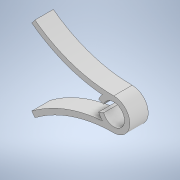
# Autodesk Inventor part: 8mmClamp
Saved by Autodesk Inventor 2020.2 (Build 242310000, 310)
## iProperties
Created: 2020-08-26
Part Number: 8mmClamp
Material: Generic
Document SubType Name: Modeling
Designer: elmar
Density: 1 g/cm^3
Appearance: Default
Author: elmar
Autodesk Inventor part; units mm, degrees
ref_plane "YZ Plane" through (0, 0, 0) normal (1, 0, 0) x (0, 1, 0)
ref_plane "XZ Plane" through (0, 0, 0) normal (0, 1, 0) x (-1, 0, 0)
ref_plane "XY Plane" through (0, 0, 0) normal (0, 0, 1) x (1, 0, 0)
sketch "Sketch1" plane through (0, 0, 0) normal (0, 0, 1) x (1, 0, 0)
  circle A0 centre (0, 0) radius 4.1
  circle A1 centre (0, 0) radius 6.1
  arc A2 (-30, 16.1) -> (0, 6.1) centre (0, 56.1) ccw
  line L0 (0, -78.54) -> (0, 78.54) projected
  arc A3 (-31.2, 14.5) -> (0, 4.1) centre (0, 56.1) ccw
  line L1 (-30, 16.1) -> (-31.2, 14.5)
  line L2 (-39.6726, 0) -> (13.7288, 0) projected
  arc A4 (0, -6.1) -> (-30, -16.1) centre (0, -56.1) ccw
  arc A5 (0, -4.1) -> (-31.2, -14.5) centre (0, -56.1) ccw
  line L3 (-30, -16.1) -> (-31.2, -14.5)
  line L4 (-5.7321, 2.0863) -> (-3.8527, 1.4023)
  line L5 (-5.7321, -2.0863) -> (-3.8527, -1.4023)
  point P0 (0, 4.1)
  point P1 (0, -4.1)
  point P2 (0, -6.1)
  point P3 (-3.8527, -1.4023)
  point P4 (-4.3447, -4.2818)
  point P5 (-4.3447, 4.2818)
  dimension "d0" = 8.2
  dimension "d1" = 2
  dimension "d3" = 50
  dimension "d4" = 30
  dimension "d7" = 20
  constraints: 10 point on circle, 8 end point, 7 symmetric about line, 5 centre point, 3 point on line, 1 coincident, 1 line through centre, 1 tangent, 6 other
  measures "d3" radius of A2
  measures "d4" horizontal distance of A1.start L1.start
  measures "d7" angle of L2 L4
extrude "Extrusion1" add sketch "Sketch1" along normal blind 7 contours L2 A1 L0 A0 | A0 L0 A1 L2 | A3 A1 L0 | A0 L4 A1 A3 | A5 A1 L5 A0 | L0 A1 A5 | A1 A3 L1 A2 | A4 L3 A5 A1
body "Solid1"
